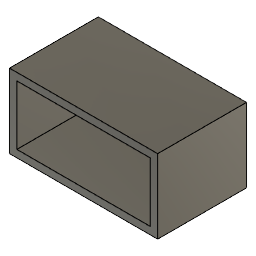
sterilization-chamber-mini (Autodesk Fusion 360 design; units mm, degrees)
part number: 2026-06-24-19-06-51-081
Autodesk Fusion 360 part; units mm, degrees
sketch "スケッチ1" plane through (0, 0, 0) normal (0, 0, 1) x (1, 0, 0)
  line L0 (0, 0) -> (-200, 0)
  line L1 (-200, 0) -> (-200, 120)
  line L2 (-200, 120) -> (0, 120)
  line L3 (0, 120) -> (0, 0)
  dimension "d1" = 200
  dimension "d2" = 120
  constraint horizontal L0
  constraint vertical L1
  constraint horizontal L2
  constraint vertical L3
  constraint coincident L0.start L3.end
  measures "d1" distance of L0.start L0.end
  measures "d2" distance of L0.start L2.end
extrude "押し出し1" add sketch "スケッチ1" along normal blind 10
sketch "スケッチ2" plane through (0, 0, 10) normal (0, 0, 1) x (-1, 0, 0)
  line L0 (0, -120) -> (200, -120)
  line L1 (200, -120) -> (200, 0)
  line L2 (200, 0) -> (0, 0)
  line L3 (0, 0) -> (0, -120)
  line L4 (190, 0) -> (190, -110)
  line L5 (190, -110) -> (10, -110)
  line L6 (10, -110) -> (10, 0)
  constraint coincident L2 L4.start
  constraint perpendicular L2 L4
  constraint perpendicular L4 L5
  constraint coincident L2 L6.end
  constraint perpendicular L2 L6
extrude "押し出し2" add sketch "スケッチ2" along normal blind 90 contours L0 L1 L2 L3 L4 L5 L6
sketch "スケッチ3" plane through (0, 110, 0) normal (0, -1, 0) x (1, 0, 0)
  line L0 (-190, 10) -> (-10, 10)
  line L1 (-10, 10) -> (-10, 100)
  line L2 (-10, 100) -> (-190, 100)
  line L3 (-190, 100) -> (-190, 10)
  line L4 (-190, 90) -> (-10, 90)
  line L5 (-10, 90) -> (-10, 100)
  line L6 (-10, 100) -> (-190, 100)
  line L7 (-190, 100) -> (-190, 90)
  constraint horizontal L4
  constraint vertical L5
  constraint horizontal L6
  constraint vertical L7
  constraint coincident L1.end L2.start
  constraint coincident L3 L4.start
extrude "押し出し3" add sketch "スケッチ3" along normal blind 110 contours L1 L2 L3 L4 L5 L6 L7
